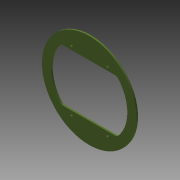
# Autodesk Inventor part: Light Sensor PCB
Saved by Autodesk Inventor 2015 (Build 190159000, 159)
## iProperties
Created: 2016-10-14
Part Number: Light Sensor PCB
Material: Generic
Document SubType Name: Modeling
Designer: James Yelland
Density: 1 g/cm^3
Appearance: Default
Author: James Yelland
Autodesk Inventor part; units mm, degrees
ref_plane "YZ Plane" through (0, 0, 0) normal (1, 0, 0) x (0, 1, 0)
ref_plane "XZ Plane" through (0, 0, 0) normal (0, 1, 0) x (-1, 0, 0)
ref_plane "XY Plane" through (0, 0, 0) normal (0, 0, 1) x (1, 0, 0)
sketch "Sketch1" plane through (0, 0, 0) normal (0, 1, 0) x (-1, 0, 0)
  circle A0 centre (0, 0) radius 59.5
  line L0 (0, 33) -> (-32.6343, 33)
  line L1 (0, 33) -> (32.6343, 33)
  line L2 (0, -33) -> (-32.6343, -33)
  line L3 (0, -33) -> (32.6343, -33)
  arc A1 (-36.429, 31.2558) -> (-36.429, -31.2558) centre (0, 0) ccw
  arc A2 (36.429, -31.2558) -> (36.429, 31.2558) centre (0, 0) ccw
  arc A3 (36.429, 31.2558) -> (32.6343, 33) centre (32.6343, 28) ccw
  arc A4 (-32.6343, 33) -> (-36.429, 31.2558) centre (-32.6343, 28) ccw
  arc A5 (-36.429, -31.2558) -> (-32.6343, -33) centre (-32.6343, -28) ccw
  arc A6 (32.6343, -33) -> (36.429, -31.2558) centre (32.6343, -28) ccw
  line L4 (32.6343, 33) -> (22.6343, 33)
  circle A7 centre (22.6343, 38) radius 1.6
  line L5 (0, 0) -> (0, 10.7969)
  line L6 (0, 0) -> (10.7386, 0)
  circle A8 centre (-22.6343, 38) radius 1.6
  circle A9 centre (22.6343, -38) radius 1.6
  circle A10 centre (-22.6343, -38) radius 1.6
  point P0 (-34.8569, 33)
  point P1 (34.8569, 33)
  point P2 (-34.8569, -33)
  point P3 (34.8569, -33)
  dimension "d1" = 119
  dimension "d7" = 5
  dimension "d8" = 10
  dimension "d11" = 3.2
  constraints: 16 point on circle, 14 end point, 11 centre point, 8 tangent, 6 point on line, 3 equal radius, 3 symmetric about line, 2 coincident, 2 horizontal, 1 vertical, 3 other
  measures "d1" diameter of A0
  measures "d7" radius of A3
  measures "d8" distance of L1.end L4.end
  measures "d11" diameter of A7
extrude "Extrusion1" add sketch "Sketch1" along normal blind 2
sketch "Sketch2" plane through (0, 0, 0) normal (0, -1, 0) x (1, 0, 0)
  line L0 (1.5, -53.75) -> (1.5, -56.75)
  line L1 (1.5, -56.75) -> (4.5, -56.75)
  line L2 (4.5, -56.75) -> (4.5, -50.75)
  line L3 (4.5, -50.75) -> (1.5, -50.75)
  line L4 (1.5, -50.75) -> (1.5, -53.75)
  line L5 (-1.5, -53.75) -> (-1.5, -56.75)
  line L6 (-1.5, -56.75) -> (-4.5, -56.75)
  line L7 (-1.5, -53.75) -> (-1.5, -53.75)
  line L8 (-1.5, -53.75) -> (-1.5, -50.75)
  line L9 (-1.5, -50.75) -> (-4.5, -50.75)
  line L10 (-4.5, -56.75) -> (-4.5, -50.75)
  line L11 (17.4817, -47.856) -> (14.584, -48.6325)
  line L12 (11.6862, -49.409) -> (8.7884, -50.1854)
  line L13 (12.4626, -52.3067) -> (11.6862, -49.409)
  line L14 (10.3413, -55.981) -> (8.7884, -50.1854)
  line L15 (14.584, -48.6325) -> (15.3604, -51.5303)
  line L16 (19.0346, -53.6516) -> (17.4817, -47.856)
  line L17 (16.1369, -54.4281) -> (19.0346, -53.6516)
  line L18 (15.3604, -51.5303) -> (16.1369, -54.4281)
  line L19 (12.4626, -52.3067) -> (13.2391, -55.2045)
  line L20 (13.2391, -55.2045) -> (10.3413, -55.981)
  line L21 (29.2721, -41.7008) -> (26.674, -43.2008)
  line L22 (24.076, -44.7008) -> (21.4779, -46.2008)
  line L23 (25.576, -47.2989) -> (24.076, -44.7008)
  line L24 (24.4779, -51.3969) -> (21.4779, -46.2008)
  line L25 (26.674, -43.2008) -> (28.174, -45.7989)
  line L26 (32.2721, -46.8969) -> (29.2721, -41.7008)
  line L27 (29.674, -48.3969) -> (32.2721, -46.8969)
  line L28 (28.174, -45.7989) -> (29.674, -48.3969)
  line L29 (25.576, -47.2989) -> (27.076, -49.8969)
  line L30 (27.076, -49.8969) -> (24.4779, -51.3969)
  line L31 (39.0676, -32.7037) -> (36.9463, -34.825)
  line L32 (34.825, -36.9463) -> (32.7037, -39.0676)
  line L33 (36.9463, -39.0676) -> (34.825, -36.9463)
  line L34 (36.9463, -43.3103) -> (32.7037, -39.0676)
  line L35 (36.9463, -34.825) -> (39.0676, -36.9463)
  line L36 (43.3103, -36.9463) -> (39.0676, -32.7037)
  line L37 (41.189, -39.0676) -> (43.3103, -36.9463)
  line L38 (39.0676, -36.9463) -> (41.189, -39.0676)
  line L39 (36.9463, -39.0676) -> (39.0676, -41.189)
  line L40 (39.0676, -41.189) -> (36.9463, -43.3103)
  line L41 (46.2008, -21.4779) -> (44.7008, -24.076)
  line L42 (43.2008, -26.674) -> (41.7008, -29.2721)
  line L43 (45.7989, -28.174) -> (43.2008, -26.674)
  line L44 (46.8969, -32.2721) -> (41.7008, -29.2721)
  line L45 (44.7008, -24.076) -> (47.2989, -25.576)
  line L46 (51.3969, -24.4779) -> (46.2008, -21.4779)
  line L47 (49.8969, -27.076) -> (51.3969, -24.4779)
  line L48 (47.2989, -25.576) -> (49.8969, -27.076)
  line L49 (45.7989, -28.174) -> (48.3969, -29.674)
  line L50 (48.3969, -29.674) -> (46.8969, -32.2721)
  line L51 (50.1854, -8.7884) -> (49.409, -11.6862)
  line L52 (48.6325, -14.584) -> (47.856, -17.4817)
  line L53 (51.5303, -15.3604) -> (48.6325, -14.584)
  line L54 (53.6516, -19.0346) -> (47.856, -17.4817)
  line L55 (49.409, -11.6862) -> (52.3067, -12.4626)
  line L56 (55.981, -10.3413) -> (50.1854, -8.7884)
  line L57 (55.2045, -13.2391) -> (55.981, -10.3413)
  line L58 (52.3067, -12.4626) -> (55.2045, -13.2391)
  line L59 (51.5303, -15.3604) -> (54.4281, -16.1369)
  line L60 (54.4281, -16.1369) -> (53.6516, -19.0346)
  line L61 (50.75, 4.5) -> (50.75, 1.5)
  line L62 (50.75, -1.5) -> (50.75, -4.5)
  line L63 (53.75, -1.5) -> (50.75, -1.5)
  line L64 (56.75, -4.5) -> (50.75, -4.5)
  line L65 (50.75, 1.5) -> (53.75, 1.5)
  line L66 (56.75, 4.5) -> (50.75, 4.5)
  line L67 (56.75, 1.5) -> (56.75, 4.5)
  line L68 (53.75, 1.5) -> (56.75, 1.5)
  line L69 (53.75, -1.5) -> (56.75, -1.5)
  line L70 (56.75, -1.5) -> (56.75, -4.5)
  line L71 (47.856, 17.4817) -> (48.6325, 14.584)
  line L72 (49.409, 11.6862) -> (50.1854, 8.7884)
  line L73 (52.3067, 12.4626) -> (49.409, 11.6862)
  line L74 (55.981, 10.3413) -> (50.1854, 8.7884)
  line L75 (48.6325, 14.584) -> (51.5303, 15.3604)
  line L76 (53.6516, 19.0346) -> (47.856, 17.4817)
  line L77 (54.4281, 16.1369) -> (53.6516, 19.0346)
  line L78 (51.5303, 15.3604) -> (54.4281, 16.1369)
  line L79 (52.3067, 12.4626) -> (55.2045, 13.2391)
  line L80 (55.2045, 13.2391) -> (55.981, 10.3413)
  line L81 (41.7008, 29.2721) -> (43.2008, 26.674)
  line L82 (44.7008, 24.076) -> (46.2008, 21.4779)
  line L83 (47.2989, 25.576) -> (44.7008, 24.076)
  line L84 (51.3969, 24.4779) -> (46.2008, 21.4779)
  line L85 (43.2008, 26.674) -> (45.7989, 28.174)
  line L86 (46.8969, 32.2721) -> (41.7008, 29.2721)
  line L87 (48.3969, 29.674) -> (46.8969, 32.2721)
  line L88 (45.7989, 28.174) -> (48.3969, 29.674)
  line L89 (47.2989, 25.576) -> (49.8969, 27.076)
  line L90 (49.8969, 27.076) -> (51.3969, 24.4779)
  line L91 (32.7037, 39.0676) -> (34.825, 36.9463)
  line L92 (36.9463, 34.825) -> (39.0676, 32.7037)
  line L93 (39.0676, 36.9463) -> (36.9463, 34.825)
  line L94 (43.3103, 36.9463) -> (39.0676, 32.7037)
  line L95 (34.825, 36.9463) -> (36.9463, 39.0676)
  line L96 (36.9463, 43.3103) -> (32.7037, 39.0676)
  line L97 (39.0676, 41.189) -> (36.9463, 43.3103)
  line L98 (36.9463, 39.0676) -> (39.0676, 41.189)
  line L99 (39.0676, 36.9463) -> (41.189, 39.0676)
  line L100 (41.189, 39.0676) -> (43.3103, 36.9463)
  line L101 (21.4779, 46.2008) -> (24.076, 44.7008)
  line L102 (26.674, 43.2008) -> (29.2721, 41.7008)
  line L103 (28.174, 45.7989) -> (26.674, 43.2008)
  line L104 (32.2721, 46.8969) -> (29.2721, 41.7008)
  line L105 (24.076, 44.7008) -> (25.576, 47.2989)
  line L106 (24.4779, 51.3969) -> (21.4779, 46.2008)
  line L107 (27.076, 49.8969) -> (24.4779, 51.3969)
  line L108 (25.576, 47.2989) -> (27.076, 49.8969)
  line L109 (28.174, 45.7989) -> (29.674, 48.3969)
  line L110 (29.674, 48.3969) -> (32.2721, 46.8969)
  line L111 (8.7884, 50.1854) -> (11.6862, 49.409)
  line L112 (14.584, 48.6325) -> (17.4817, 47.856)
  line L113 (15.3604, 51.5303) -> (14.584, 48.6325)
  line L114 (19.0346, 53.6516) -> (17.4817, 47.856)
  line L115 (11.6862, 49.409) -> (12.4626, 52.3067)
  line L116 (10.3413, 55.981) -> (8.7884, 50.1854)
  line L117 (13.2391, 55.2045) -> (10.3413, 55.981)
  line L118 (12.4626, 52.3067) -> (13.2391, 55.2045)
  line L119 (15.3604, 51.5303) -> (16.1369, 54.4281)
  line L120 (16.1369, 54.4281) -> (19.0346, 53.6516)
  line L121 (-4.5, 50.75) -> (-1.5, 50.75)
  line L122 (1.5, 50.75) -> (4.5, 50.75)
  line L123 (1.5, 53.75) -> (1.5, 50.75)
  line L124 (4.5, 56.75) -> (4.5, 50.75)
  line L125 (-1.5, 50.75) -> (-1.5, 53.75)
  line L126 (-4.5, 56.75) -> (-4.5, 50.75)
  line L127 (-1.5, 56.75) -> (-4.5, 56.75)
  line L128 (-1.5, 53.75) -> (-1.5, 56.75)
  line L129 (1.5, 53.75) -> (1.5, 56.75)
  line L130 (1.5, 56.75) -> (4.5, 56.75)
  line L131 (-17.4817, 47.856) -> (-14.584, 48.6325)
  line L132 (-11.6862, 49.409) -> (-8.7884, 50.1854)
  line L133 (-12.4626, 52.3067) -> (-11.6862, 49.409)
  line L134 (-10.3413, 55.981) -> (-8.7884, 50.1854)
  line L135 (-14.584, 48.6325) -> (-15.3604, 51.5303)
  line L136 (-19.0346, 53.6516) -> (-17.4817, 47.856)
  line L137 (-16.1369, 54.4281) -> (-19.0346, 53.6516)
  line L138 (-15.3604, 51.5303) -> (-16.1369, 54.4281)
  line L139 (-12.4626, 52.3067) -> (-13.2391, 55.2045)
  line L140 (-13.2391, 55.2045) -> (-10.3413, 55.981)
  line L141 (-29.2721, 41.7008) -> (-26.674, 43.2008)
  line L142 (-24.076, 44.7008) -> (-21.4779, 46.2008)
  line L143 (-25.576, 47.2989) -> (-24.076, 44.7008)
  line L144 (-24.4779, 51.3969) -> (-21.4779, 46.2008)
  line L145 (-26.674, 43.2008) -> (-28.174, 45.7989)
  line L146 (-32.2721, 46.8969) -> (-29.2721, 41.7008)
  line L147 (-29.674, 48.3969) -> (-32.2721, 46.8969)
  line L148 (-28.174, 45.7989) -> (-29.674, 48.3969)
  line L149 (-25.576, 47.2989) -> (-27.076, 49.8969)
  line L150 (-27.076, 49.8969) -> (-24.4779, 51.3969)
  line L151 (-39.0676, 32.7037) -> (-36.9463, 34.825)
  line L152 (-34.825, 36.9463) -> (-32.7037, 39.0676)
  line L153 (-36.9463, 39.0676) -> (-34.825, 36.9463)
  line L154 (-36.9463, 43.3103) -> (-32.7037, 39.0676)
  line L155 (-36.9463, 34.825) -> (-39.0676, 36.9463)
  line L156 (-43.3103, 36.9463) -> (-39.0676, 32.7037)
  line L157 (-41.189, 39.0676) -> (-43.3103, 36.9463)
  line L158 (-39.0676, 36.9463) -> (-41.189, 39.0676)
  line L159 (-36.9463, 39.0676) -> (-39.0676, 41.189)
  line L160 (-39.0676, 41.189) -> (-36.9463, 43.3103)
  line L161 (-46.2008, 21.4779) -> (-44.7008, 24.076)
  line L162 (-43.2008, 26.674) -> (-41.7008, 29.2721)
  line L163 (-45.7989, 28.174) -> (-43.2008, 26.674)
  line L164 (-46.8969, 32.2721) -> (-41.7008, 29.2721)
  line L165 (-44.7008, 24.076) -> (-47.2989, 25.576)
  line L166 (-51.3969, 24.4779) -> (-46.2008, 21.4779)
  line L167 (-49.8969, 27.076) -> (-51.3969, 24.4779)
  line L168 (-47.2989, 25.576) -> (-49.8969, 27.076)
  line L169 (-45.7989, 28.174) -> (-48.3969, 29.674)
  line L170 (-48.3969, 29.674) -> (-46.8969, 32.2721)
  line L171 (-50.1854, 8.7884) -> (-49.409, 11.6862)
  line L172 (-48.6325, 14.584) -> (-47.856, 17.4817)
  line L173 (-51.5303, 15.3604) -> (-48.6325, 14.584)
  line L174 (-53.6516, 19.0346) -> (-47.856, 17.4817)
  line L175 (-49.409, 11.6862) -> (-52.3067, 12.4626)
  line L176 (-55.981, 10.3413) -> (-50.1854, 8.7884)
  line L177 (-55.2045, 13.2391) -> (-55.981, 10.3413)
  line L178 (-52.3067, 12.4626) -> (-55.2045, 13.2391)
  line L179 (-51.5303, 15.3604) -> (-54.4281, 16.1369)
  line L180 (-54.4281, 16.1369) -> (-53.6516, 19.0346)
  line L181 (-50.75, -4.5) -> (-50.75, -1.5)
  line L182 (-50.75, 1.5) -> (-50.75, 4.5)
  line L183 (-53.75, 1.5) -> (-50.75, 1.5)
  line L184 (-56.75, 4.5) -> (-50.75, 4.5)
  line L185 (-50.75, -1.5) -> (-53.75, -1.5)
  line L186 (-56.75, -4.5) -> (-50.75, -4.5)
  line L187 (-56.75, -1.5) -> (-56.75, -4.5)
  line L188 (-53.75, -1.5) -> (-56.75, -1.5)
  line L189 (-53.75, 1.5) -> (-56.75, 1.5)
  line L190 (-56.75, 1.5) -> (-56.75, 4.5)
  line L191 (-47.856, -17.4817) -> (-48.6325, -14.584)
  line L192 (-49.409, -11.6862) -> (-50.1854, -8.7884)
  line L193 (-52.3067, -12.4626) -> (-49.409, -11.6862)
  line L194 (-55.981, -10.3413) -> (-50.1854, -8.7884)
  line L195 (-48.6325, -14.584) -> (-51.5303, -15.3604)
  line L196 (-53.6516, -19.0346) -> (-47.856, -17.4817)
  line L197 (-54.4281, -16.1369) -> (-53.6516, -19.0346)
  line L198 (-51.5303, -15.3604) -> (-54.4281, -16.1369)
  line L199 (-52.3067, -12.4626) -> (-55.2045, -13.2391)
  line L200 (-55.2045, -13.2391) -> (-55.981, -10.3413)
  line L201 (-41.7008, -29.2721) -> (-43.2008, -26.674)
  line L202 (-44.7008, -24.076) -> (-46.2008, -21.4779)
  line L203 (-47.2989, -25.576) -> (-44.7008, -24.076)
  line L204 (-51.3969, -24.4779) -> (-46.2008, -21.4779)
  line L205 (-43.2008, -26.674) -> (-45.7989, -28.174)
  line L206 (-46.8969, -32.2721) -> (-41.7008, -29.2721)
  line L207 (-48.3969, -29.674) -> (-46.8969, -32.2721)
  line L208 (-45.7989, -28.174) -> (-48.3969, -29.674)
  line L209 (-47.2989, -25.576) -> (-49.8969, -27.076)
  line L210 (-49.8969, -27.076) -> (-51.3969, -24.4779)
  line L211 (-32.7037, -39.0676) -> (-34.825, -36.9463)
  line L212 (-36.9463, -34.825) -> (-39.0676, -32.7037)
  line L213 (-39.0676, -36.9463) -> (-36.9463, -34.825)
  line L214 (-43.3103, -36.9463) -> (-39.0676, -32.7037)
  line L215 (-34.825, -36.9463) -> (-36.9463, -39.0676)
  line L216 (-36.9463, -43.3103) -> (-32.7037, -39.0676)
  line L217 (-39.0676, -41.189) -> (-36.9463, -43.3103)
  line L218 (-36.9463, -39.0676) -> (-39.0676, -41.189)
  line L219 (-39.0676, -36.9463) -> (-41.189, -39.0676)
  line L220 (-41.189, -39.0676) -> (-43.3103, -36.9463)
  line L221 (-21.4779, -46.2008) -> (-24.076, -44.7008)
  line L222 (-26.674, -43.2008) -> (-29.2721, -41.7008)
  line L223 (-28.174, -45.7989) -> (-26.674, -43.2008)
  line L224 (-32.2721, -46.8969) -> (-29.2721, -41.7008)
  line L225 (-24.076, -44.7008) -> (-25.576, -47.2989)
  line L226 (-24.4779, -51.3969) -> (-21.4779, -46.2008)
  line L227 (-27.076, -49.8969) -> (-24.4779, -51.3969)
  line L228 (-25.576, -47.2989) -> (-27.076, -49.8969)
  line L229 (-28.174, -45.7989) -> (-29.674, -48.3969)
  line L230 (-29.674, -48.3969) -> (-32.2721, -46.8969)
  line L231 (-8.7884, -50.1854) -> (-11.6862, -49.409)
  line L232 (-14.584, -48.6325) -> (-17.4817, -47.856)
  line L233 (-15.3604, -51.5303) -> (-14.584, -48.6325)
  line L234 (-19.0346, -53.6516) -> (-17.4817, -47.856)
  line L235 (-11.6862, -49.409) -> (-12.4626, -52.3067)
  line L236 (-10.3413, -55.981) -> (-8.7884, -50.1854)
  line L237 (-13.2391, -55.2045) -> (-10.3413, -55.981)
  line L238 (-12.4626, -52.3067) -> (-13.2391, -55.2045)
  line L239 (-15.3604, -51.5303) -> (-16.1369, -54.4281)
  line L240 (-16.1369, -54.4281) -> (-19.0346, -53.6516)
  line L241 (-32.6343, 33) -> (32.6343, 33) projected
  arc A0 (36.429, 31.2558) -> (32.6343, 33) centre (32.6343, 28) ccw projected
  arc A1 (36.429, -31.2558) -> (36.429, 31.2558) centre (0, 0) ccw projected
  arc A2 (32.6343, -33) -> (36.429, -31.2558) centre (32.6343, -28) ccw projected
  line L242 (32.6343, -33) -> (-32.6343, -33) projected
  arc A3 (-36.429, -31.2558) -> (-32.6343, -33) centre (-32.6343, -28) ccw projected
  arc A4 (-36.429, 31.2558) -> (-36.429, -31.2558) centre (0, 0) ccw projected
  arc A5 (-32.6343, 33) -> (-36.429, 31.2558) centre (-32.6343, 28) ccw projected
  circle A6 centre (-22.6343, -38) radius 1.6 projected
  circle A7 centre (22.6343, -38) radius 1.6 projected
  circle A8 centre (22.6343, 38) radius 1.6 projected
  circle A9 centre (-22.6343, 38) radius 1.6 projected
  circle A10 centre (0, 0) radius 59.5 projected
  constraints: 482 end point, 24 point on line, 2 coincident
sketch "Sketch3" plane through (0, 2, 0) normal (0, 1, 0) x (1, 0, 0)
  line L0 (-86.7436, 84.5991) -> (77.9188, 84.5991) construction
  line L1 (77.9188, 84.5991) -> (77.9188, -81.7059) construction
  line L2 (77.9188, -81.7059) -> (-86.7436, -81.7059) construction
  line L3 (-86.7436, -81.7059) -> (-86.7436, 84.5991) construction
  line L4 (32.6343, -33) -> (-32.6343, -33) projected
  arc A0 (-36.429, -31.2558) -> (-32.6343, -33) centre (-32.6343, -28) ccw projected
  arc A1 (-36.429, 31.2558) -> (-36.429, -31.2558) centre (0, 0) ccw projected
  arc A2 (-32.6343, 33) -> (-36.429, 31.2558) centre (-32.6343, 28) ccw projected
  line L5 (-32.6343, 33) -> (32.6343, 33) projected
  arc A3 (36.429, 31.2558) -> (32.6343, 33) centre (32.6343, 28) ccw projected
  arc A4 (36.429, -31.2558) -> (36.429, 31.2558) centre (0, 0) ccw projected
  arc A5 (32.6343, -33) -> (36.429, -31.2558) centre (32.6343, -28) ccw projected
  circle A6 centre (-22.6343, 38) radius 1.6 projected
  circle A7 centre (22.6343, 38) radius 1.6 projected
  circle A8 centre (22.6343, -38) radius 1.6 projected
  circle A9 centre (-22.6343, -38) radius 1.6 projected
  circle A10 centre (0, 0) radius 59.5 projected
  constraints: 2 other
decal "Decal1"
body "Solid1"
